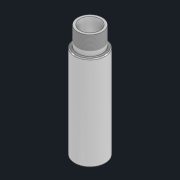
# Autodesk Inventor part: EndHilt
Saved by Autodesk Inventor 2022.1 (Build 261234000, 234)
## iProperties
Created: 2022-01-30
Part Number: EndHilt
Material: Aluminum 6061
Document SubType Name: Modeling
Designer: Michael Lacey
Mass: 279.361 g
Surface Area: 334.581 cm^2
Volume: 103.467 cm^3
Density: 2.7 g/cm^3
Appearance: Aluminum - Flat
Author: Michael Lacey
Autodesk Inventor part; units mm, degrees
ref_plane "YZ Plane" through (0, 0, 0) normal (1, 0, 0) x (0, 1, 0)
ref_plane "XZ Plane" through (0, 0, 0) normal (0, 1, 0) x (-1, 0, 0)
ref_plane "XY Plane" through (0, 0, 0) normal (0, 0, 1) x (1, 0, 0)
sketch "Sketch1" plane through (0, 0, 0) normal (0, 1, 0) x (-1, 0, 0)
  line L0 (0, 74.2932) -> (20.6375, 74.2932)
  line L1 (20.6375, 74.2932) -> (20.6375, 45.7421)
  line L2 (13.589, 67.9432) -> (0, 67.9432)
  line L3 (16.6624, -52.7068) -> (20.6375, -52.7068)
  line L4 (20.6375, -52.7068) -> (20.6375, 45.7421)
  line L5 (16.6624, -52.7068) -> (16.6624, -78.1068)
  line L6 (16.6624, -78.1068) -> (13.589, -78.1068)
  line L7 (13.589, -78.1068) -> (13.589, 67.9432)
  line L8 (0, 68.4776) -> (0, -51.9613) construction
  line L9 (13.589, 67.9432) -> (13.589, 74.2932)
  point P0 (0, 0)
  dimension "d0" = 20.6375
  dimension "d1" = 127
  dimension "d2" = 6.35
  dimension "d3" = 16.6624
  dimension "d4" = 13.589
  dimension "d12" = 25.4
  dimension "d19" = 3.0734
  constraints: 20 end point, 3 point on line, 2 parallel, 2 perpendicular, 1 horizontal, 1 vertical
  measures "d0" distance from line of L1.end L8
  measures "d1" distance between parallel lines of L3 L0
  measures "d2" distance between parallel lines of L0 L2
  measures "d3" distance between parallel lines of L8 L5
  measures "d4" distance between parallel lines of L8 L7
  measures "d12" distance between parallel lines of L6 L3
  measures "d19" distance between parallel lines of L7 L5
revolve "Revolution1" add sketch "Sketch1" angle 360 about axis through (0, 0, 68.4776) along (0, 0, -1)
thread "Thread1" size "1 5/16-18 UNEF" class "2A" standard "ANSI Unified Screw Threads" length 19.05
chamfer "Chamfer2" distance 1.27 angle 45 1 edges at (20.6375, 0, -52.7068)
chamfer "Chamfer3" distance 1.27 angle 45 1 edges at (20.6375, 0, 74.2932)
body "Solid1"
